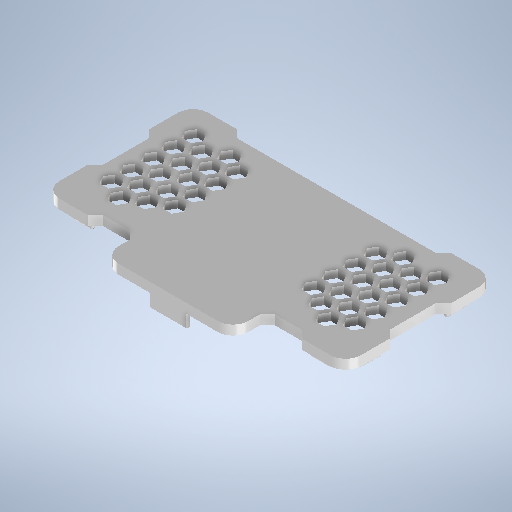
# Autodesk Inventor part: untitled22223333
Saved by Autodesk Inventor 2025.2 (Build 292293000, 293)
## iProperties
Created: 2025-03-09
Part Number: untitled22223333
Material: Ogólny
Document SubType Name: Modeling
Designer: admin
Density: 1 g/cm^3
Appearance: Domyślna
Author: admin
Autodesk Inventor part; units mm, degrees
(part 1 of 3)
ref_plane "YZ Plane" through (0, 0, 0) normal (1, 0, 0) x (0, 1, 0)
ref_plane "XZ Plane" through (0, 0, 0) normal (0, 1, 0) x (-1, 0, 0)
sketch "Szkic1" plane through (0, 0, 0) normal (0, 0, 1) x (1, 0, 0)
  line L0 (-39.2454, 11.2956) -> (-39.2454, -13.7044)
  line L1 (-36.2454, -16.7044) -> (28.7546, -16.7044)
  line L2 (31.7546, -13.7044) -> (31.7546, 11.2956)
  line L3 (-41.2454, 4.7956) -> (-41.2454, -7.2044)
  line L4 (-29.7595, -18.7044) -> (22.2546, -18.7044)
  line L5 (33.7546, -7.2044) -> (33.7546, 4.7956)
  line L6 (-43.2454, -9.2044) -> (-43.2454, -9.2044)
  line L7 (-43.2454, 6.7956) -> (-43.2454, 6.7956)
  line L8 (-39.2454, 6.7956) -> (-39.2454, -9.2044)
  line L9 (35.7546, -9.2044) -> (35.7546, -9.2044)
  line L10 (35.7546, 6.7956) -> (35.7546, 6.7956)
  line L11 (31.7546, 6.7956) -> (31.7546, -9.2044)
  line L12 (35.7546, 14.2956) -> (35.7546, 6.7956)
  line L13 (35.7546, -9.2044) -> (35.7546, -16.7044)
  line L14 (-43.2454, -16.7044) -> (-43.2454, -9.2044)
  line L15 (-43.2454, 6.7956) -> (-43.2454, 14.2956)
  line L16 (-31.7454, -20.7044) -> (-31.7454, -20.7044)
  line L17 (24.2546, -20.7044) -> (24.2546, -20.7044)
  line L18 (24.2546, 18.2956) -> (24.2546, 18.2956)
  line L19 (-31.7454, 18.2956) -> (-31.7454, 18.2956)
  line L20 (-39.2454, 18.2956) -> (-31.7454, 18.2956)
  line L21 (24.2546, 18.2956) -> (31.7546, 18.2956)
  line L22 (31.7546, -20.7044) -> (24.2546, -20.7044)
  line L23 (-31.7454, -20.7044) -> (-39.2454, -20.7044)
  line L24 (-31.7454, 18.2956) -> (-29.7454, 16.2956)
  line L25 (-43.2454, 6.7956) -> (-41.2454, 4.7956)
  line L26 (-43.2454, -9.2044) -> (-41.2454, -7.2044)
  line L27 (-31.7454, -20.7044) -> (-29.7595, -18.7044)
  line L28 (22.2546, -18.7044) -> (24.2546, -20.7044)
  line L29 (35.7546, -9.2044) -> (33.7546, -7.2044)
  line L30 (35.7546, 6.7956) -> (33.7546, 4.7956)
  line L31 (24.2546, 18.2956) -> (22.2546, 16.2956)
  line L32 (22.2546, 16.2956) -> (15.2546, 16.2956)
  line L33 (-22.7454, 16.2956) -> (-29.7454, 16.2956)
  arc A0 (-39.2454, 18.2956) -> (-43.2454, 14.2956) centre (-39.2454, 14.2956) ccw
  arc A1 (-43.2454, -16.7044) -> (-39.2454, -20.7044) centre (-39.2454, -16.7044) ccw
  arc A2 (31.7546, -20.7044) -> (35.7546, -16.7044) centre (31.7546, -16.7044) ccw
  arc A3 (35.7546, 14.2956) -> (31.7546, 18.2956) centre (31.7546, 14.2956) ccw
  line L34 (13.2546, 18.2956) -> (13.2546, 21.2956)
  line L35 (6.2546, 24.2956) -> (-13.7454, 24.2956)
  line L36 (-20.7454, 21.2956) -> (-20.7454, 18.2956)
  line L37 (-16.7454, 16.2956) -> (-16.7454, 21.2956)
  line L38 (9.2546, 16.2956) -> (9.2546, 21.2956)
  line L39 (13.2546, 18.2956) -> (15.2546, 16.2956)
  line L40 (-20.7454, 18.2956) -> (-22.7454, 16.2956)
  line L41 (-36.2454, 14.2956) -> (-19.5739, 14.2956)
  line L42 (-13.917, 24.2956) -> (6.4261, 24.2956)
  line L43 (9.2546, 25.2956) -> (-16.7454, 25.2956)
  arc A4 (-16.7454, 25.2956) -> (-20.7454, 21.2956) centre (-16.7454, 21.2956) ccw
  arc A5 (13.2546, 21.2956) -> (9.2546, 25.2956) centre (9.2546, 21.2956) ccw
  arc A6 (31.7546, 11.2956) -> (28.7546, 14.2956) centre (28.7546, 11.2956) ccw
  arc A7 (28.7546, -16.7044) -> (31.7546, -13.7044) centre (28.7546, -13.7044) ccw
  arc A8 (-39.2454, -13.7044) -> (-36.2454, -16.7044) centre (-36.2454, -13.7044) ccw
  arc A9 (-36.2454, 14.2956) -> (-39.2454, 11.2956) centre (-36.2454, 11.2956) ccw
  arc A10 (-13.7454, 24.2956) -> (-16.7454, 21.2956) centre (-13.7454, 21.2956) ccw
  arc A11 (9.2546, 21.2956) -> (6.2546, 24.2956) centre (6.2546, 21.2956) ccw
  line L44 (28.7546, 14.2956) -> (11.2546, 14.2956)
  line L45 (-18.7454, 14.2956) -> (-19.5739, 14.2956)
  arc A12 (-18.7454, 14.2956) -> (-16.7454, 16.2956) centre (-18.7454, 16.2956) ccw
  arc A13 (9.2546, 16.2956) -> (11.2546, 14.2956) centre (11.2546, 16.2956) ccw
  line L46 (-31.7454, -18.7044) -> (-38.2454, -18.7044) construction
  line L47 (-32.6454, -17.8044) -> (-37.3454, -17.8044)
  line L48 (-37.3454, -19.6044) -> (-32.6454, -19.6044)
  arc A14 (-32.6454, -19.6044) -> (-32.6454, -17.8044) centre (-32.6454, -18.7044) ccw
  arc A15 (-37.3454, -17.8044) -> (-37.3454, -19.6044) centre (-37.3454, -18.7044) ccw
  line L49 (-41.2454, -9.2044) -> (-41.2454, -15.7044) construction
  line L50 (-42.1454, -10.1044) -> (-42.1454, -14.8044)
  line L51 (-40.3454, -14.8044) -> (-40.3454, -10.1044)
  arc A16 (-40.3454, -10.1044) -> (-42.1454, -10.1044) centre (-41.2454, -10.1044) ccw
  arc A17 (-42.1454, -14.8044) -> (-40.3454, -14.8044) centre (-41.2454, -14.8044) ccw
  circle A18 centre (-40.2454, -17.7044) radius 1.5
  line L52 (24.2546, -18.7044) -> (30.7546, -18.7044) construction
  line L53 (25.1546, -17.8044) -> (29.8546, -17.8044)
  line L54 (29.8546, -19.6044) -> (25.1546, -19.6044)
  arc A19 (25.1546, -17.8044) -> (25.1546, -19.6044) centre (25.1546, -18.7044) ccw
  arc A20 (29.8546, -19.6044) -> (29.8546, -17.8044) centre (29.8546, -18.7044) ccw
  line L55 (33.7546, -9.2044) -> (33.7546, -15.7044) construction
  line L56 (34.6546, -10.1044) -> (34.6546, -14.8044)
  line L57 (32.8546, -14.8044) -> (32.8546, -10.1044)
  arc A21 (34.6546, -10.1044) -> (32.8546, -10.1044) centre (33.7546, -10.1044) ccw
  arc A22 (32.8546, -14.8044) -> (34.6546, -14.8044) centre (33.7546, -14.8044) ccw
  circle A23 centre (32.7546, -17.7044) radius 1.5
  line L58 (-43.2454, 6.7956) -> (-41.2454, 4.7956)
  line L59 (-31.7454, 16.2956) -> (-38.2454, 16.2956) construction
  line L60 (-32.6454, 15.3956) -> (-37.3454, 15.3956)
  line L61 (-37.3454, 17.1956) -> (-32.6454, 17.1956)
  arc A24 (-32.6454, 15.3956) -> (-32.6454, 17.1956) centre (-32.6454, 16.2956) ccw
  arc A25 (-37.3454, 17.1956) -> (-37.3454, 15.3956) centre (-37.3454, 16.2956) ccw
  line L62 (-41.2454, 6.7956) -> (-41.2454, 13.2956) construction
  line L63 (-42.1454, 7.6956) -> (-42.1454, 12.3956)
  line L64 (-40.3454, 12.3956) -> (-40.3454, 7.6956)
  arc A26 (-42.1454, 7.6956) -> (-40.3454, 7.6956) centre (-41.2454, 7.6956) ccw
  arc A27 (-40.3454, 12.3956) -> (-42.1454, 12.3956) centre (-41.2454, 12.3956) ccw
  circle A28 centre (-40.2454, 15.2956) radius 1.5
  circle A29 centre (32.7546, 15.2956) radius 1.5
  arc A30 (32.8546, 7.6956) -> (34.6546, 7.6956) centre (33.7546, 7.6956) ccw
  line L65 (34.6546, 7.6956) -> (34.6546, 12.3956)
  line L66 (33.7546, 6.7956) -> (33.7546, 13.2956) construction
  arc A31 (34.6546, 12.3956) -> (32.8546, 12.3956) centre (33.7546, 12.3956) ccw
  line L67 (32.8546, 12.3956) -> (32.8546, 7.6956)
  line L68 (24.2546, 16.2956) -> (30.7546, 16.2956) construction
  arc A32 (29.8546, 15.3956) -> (29.8546, 17.1956) centre (29.8546, 16.2956) ccw
  line L69 (29.8546, 17.1956) -> (25.1546, 17.1956)
  arc A33 (25.1546, 17.1956) -> (25.1546, 15.3956) centre (25.1546, 16.2956) ccw
  line L70 (25.1546, 15.3956) -> (29.8546, 15.3956)
  point P0 (0, 0)
  point P1 (33.7546, 6.7956)
  point P2 (-31.7454, 16.2956)
  point P3 (24.2546, -18.7044)
  point P4 (24.2546, 16.2956)
  point P5 (33.7546, -9.2044)
  point P6 (-41.2454, 6.7956)
  point P7 (-20.7454, 16.2956)
  point P8 (13.2546, 16.2956)
  point P9 (-16.7454, 24.2956)
  point P10 (24.2546, -20.7044)
  point P11 (35.7546, 6.7956)
  point P12 (24.2546, 18.2956)
  point P13 (-43.2454, 6.7956)
  point P14 (-34.9954, -18.7044)
  point P15 (-41.2454, -12.4544)
  point P16 (27.5046, -18.7044)
  point P17 (33.7546, -12.4544)
  point P18 (24.2546, 16.2956)
  point P19 (33.7546, 6.7956)
  point P20 (-34.9954, 16.2956)
  point P21 (-41.2454, 10.0456)
  point P22 (33.7546, 10.0456)
  point P23 (27.5046, 16.2956)
  dimension "d0" = 4
  dimension "d2" = 3
  dimension "d3" = 2
  dimension "d17" = 6.5
  dimension "d18" = 1.8
  dimension "d19" = 6.5
  dimension "d20" = 1.8
  dimension "d23" = 3
  dimension "d81" = 3
  dimension "d82" = 3
  dimension "d83" = 3
  constraints: 158 end point, 76 point on circle, 40 point on line, 37 tangent, 34 centre point, 25 parallel, 9 perpendicular, 8 equal radius, 4 horizontal, 2 midpoint, 1 vertical
  measures "d0" radius of A0
  measures "d2" radius of A10
  measures "d3" radius of A12
  measures "d17" distance of L46.start L46.end
  measures "d18" diameter of A15
  measures "d19" distance of L49.start L49.end
  measures "d20" diameter of A17
  measures "d23" diameter of A18
  measures "d81" diameter of A28
  measures "d82" diameter of A29
  measures "d83" diameter of A23
extrude "Wyciągnięcie proste1" add sketch "Szkic1" along normal blind 2.5 contours A9 L41 L45 A12 L37 A10 L35 A11 L38 A13 L44 A6 L2 A7 L1 A8 L0 | L25 L15 A0 L20 L24 L33 L40 L36 A4 L43 A5 L34 L39 L32 L31 L21 A3 L12 L30 L5 L29 L13 A2 L22 L28 L4 L27 L23 A1 L14 L26 L3 | A14 L48 A15 L47 | A16 L51 A17 L50 | A18 | L53 A20 L54 A19 | L56 A22 L57 A21 | A23 | L60 A25 L61 A24 | L63 A27 L64 A26 | A28 | A29 | L67 A31 L65 A30 | L70 A33 L69 A32
extrude "Wyciągnięcie proste4" cut sketch "Szkic1" along normal blind 1.6 contours A18 | A23 | A28 | A29
sketch "Szkic4" plane through (0, 0, 0) normal (0, 0, -1) x (-1, 0, 0)
  line L0 (-9.2546, 25.2956) -> (16.7454, 25.2956) projected
  line L1 (-0.9446, 24.2956) -> (8.4354, 24.2956)
  line L2 (8.4354, 24.2956) -> (8.4354, 25.2956)
  line L3 (8.4354, 26.2956) -> (-0.9446, 24.2956) construction
  line L4 (-0.9446, 26.2956) -> (8.4354, 24.2956) construction
  line L5 (8.4354, 25.2956) -> (-0.9446, 25.2956)
  line L6 (-0.9446, 24.2956) -> (-0.9446, 25.2956)
  line L7 (8.4354, 25.2956) -> (-0.9446, 25.2956)
  point P0 (0, 0)
  constraints: 14 end point, 1 collinear, 1 perpendicular, 1 point on line
extrude "Wyciągnięcie proste6" add sketch "Szkic4" along normal blind 3.5
sketch "Szkic5" plane through (0, 0, 0) normal (0, 0, -1) x (-1, 0, 0)
  line L0 (8.4425, -20.7044) -> (-0.9375, -20.7044)
  line L1 (-0.9375, -20.7044) -> (-0.9375, -16.7044)
  line L2 (-0.9375, -16.7044) -> (8.4425, -16.7044)
  line L3 (8.4425, -16.7044) -> (8.4425, -20.7044)
  line L4 (29.7595, -18.7044) -> (-22.2546, -18.7044) projected
  line L5 (8.4425, -20.7044) -> (-0.9375, -16.7044) construction
  line L6 (-0.9375, -20.7044) -> (8.4425, -16.7044) construction
  line L7 (8.4425, -18.7044) -> (-0.9375, -18.7044)
  point P0 (0, 0)
  point P1 (3.7525, -18.7044)
  dimension "d32" = 9.38
  dimension "d33" = 4
  constraints: 14 end point, 5 midpoint, 2 parallel, 2 point on line, 1 horizontal, 1 perpendicular
  measures "d32" distance of L1.end L2.end
  measures "d33" distance of L0.end L1.end
extrude "Wyciągnięcie proste7" add sketch "Szkic5" along normal blind 4 contours L4 L1 L2 L3
ref_plane "Płaszczyzna konstrukcyjna2" through (0, 0, -2) normal (0, 0, -1) x (-1, 0, 0)
sketch "Szkic7" plane through (0, 0, -2) normal (0, 0, -1) x (-1, 0, 0)
  arc A0 (-25.1546, 15.6456) -> (-25.1546, 16.9456) centre (-25.1546, 16.2956) ccw projected
  arc A1 (-29.8546, 16.9456) -> (-29.8546, 15.6456) centre (-29.8546, 16.2956) ccw projected
  line L0 (-25.1546, 16.2956) -> (-25.2546, 16.2956)
  line L1 (-29.8546, 16.2956) -> (-29.7546, 16.2956)
  arc A2 (-25.2546, 15.3956) -> (-25.2546, 17.1956) centre (-25.2546, 16.2956) ccw
  line L2 (-25.1546, 15.3956) -> (-29.8546, 15.3956) projected
  arc A3 (-29.7546, 17.1956) -> (-29.7546, 15.3956) centre (-29.7546, 16.2956) ccw
  line L3 (-25.2546, 15.3956) -> (-29.7546, 15.3956)
  line L4 (-25.2546, 17.1956) -> (-29.7546, 17.1956)
  line L5 (-25.1546, 17.1956) -> (-29.8546, 17.1956) projected
  line L6 (-33.7546, 12.3956) -> (-33.7546, 12.2956)
  arc A4 (-34.4046, 7.6956) -> (-33.1046, 7.6956) centre (-33.7546, 7.6956) ccw projected
  line L7 (-33.7546, 7.6956) -> (-33.7546, 7.7956)
  arc A5 (-32.8546, 12.2956) -> (-34.6546, 12.2956) centre (-33.7546, 12.2956) ccw
  line L8 (-34.6546, 7.6956) -> (-34.6546, 12.3956) projected
  arc A6 (-34.6546, 7.7956) -> (-32.8546, 7.7956) centre (-33.7546, 7.7956) ccw
  line L9 (-32.8546, 12.3956) -> (-32.8546, 7.6956) projected
  line L10 (-32.8546, 7.7956) -> (-32.8546, 12.2956)
  line L11 (-34.6546, 12.2956) -> (-34.6546, 7.7956)
  line L12 (-33.7546, -7.2044) -> (-33.7546, 4.7956) projected
  line L13 (-33.7546, -1.2044) -> (-29.2219, -1.2044)
  line L14 (8.4354, 25.2956) -> (-0.9446, 25.2956) projected
  line L15 (3.7454, 25.2956) -> (3.7454, 21.1708)
  arc A7 (-25.1546, -19.3544) -> (-25.1546, -18.0544) centre (-25.1546, -18.7044) ccw
  arc A8 (-29.8546, -18.0544) -> (-29.8546, -19.3544) centre (-29.8546, -18.7044) ccw
  line L16 (-25.1546, -18.7044) -> (-25.2546, -18.7044)
  line L17 (-29.8546, -18.7044) -> (-29.7546, -18.7044)
  arc A9 (-25.2546, -19.6044) -> (-25.2546, -17.8044) centre (-25.2546, -18.7044) ccw
  line L18 (-25.1546, -17.8044) -> (-29.8546, -17.8044)
  arc A10 (-29.7546, -17.8044) -> (-29.7546, -19.6044) centre (-29.7546, -18.7044) ccw
  line L19 (-25.2546, -17.8044) -> (-29.7546, -17.8044)
  line L20 (-25.2546, -19.6044) -> (-29.7546, -19.6044)
  line L21 (-25.1546, -19.6044) -> (-29.8546, -19.6044)
  line L22 (-33.7546, -14.8044) -> (-33.7546, -14.7044)
  arc A11 (-33.1046, -10.1044) -> (-34.4046, -10.1044) centre (-33.7546, -10.1044) ccw
  line L23 (-33.7546, -10.1044) -> (-33.7546, -10.2044)
  arc A12 (-34.6546, -14.7044) -> (-32.8546, -14.7044) centre (-33.7546, -14.7044) ccw
  line L24 (-34.6546, -10.1044) -> (-34.6546, -14.8044)
  arc A13 (-32.8546, -10.2044) -> (-34.6546, -10.2044) centre (-33.7546, -10.2044) ccw
  line L25 (-32.8546, -14.8044) -> (-32.8546, -10.1044)
  line L26 (-32.8546, -10.2044) -> (-32.8546, -14.7044)
  line L27 (-34.6546, -14.7044) -> (-34.6546, -10.2044)
  arc A14 (32.6454, 16.9456) -> (32.6454, 15.6456) centre (32.6454, 16.2956) ccw
  arc A15 (37.3454, 15.6456) -> (37.3454, 16.9456) centre (37.3454, 16.2956) ccw
  line L28 (32.6454, 16.2956) -> (32.7454, 16.2956)
  line L29 (37.3454, 16.2956) -> (37.2454, 16.2956)
  arc A16 (32.7454, 17.1956) -> (32.7454, 15.3956) centre (32.7454, 16.2956) ccw
  line L30 (32.6454, 15.3956) -> (37.3454, 15.3956)
  arc A17 (37.2454, 15.3956) -> (37.2454, 17.1956) centre (37.2454, 16.2956) ccw
  line L31 (32.7454, 15.3956) -> (37.2454, 15.3956)
  line L32 (32.7454, 17.1956) -> (37.2454, 17.1956)
  line L33 (32.6454, 17.1956) -> (37.3454, 17.1956)
  line L34 (41.2454, 12.3956) -> (41.2454, 12.2956)
  arc A18 (40.5954, 7.6956) -> (41.8954, 7.6956) centre (41.2454, 7.6956) ccw
  line L35 (41.2454, 7.6956) -> (41.2454, 7.7956)
  arc A19 (42.1454, 12.2956) -> (40.3454, 12.2956) centre (41.2454, 12.2956) ccw
  line L36 (42.1454, 7.6956) -> (42.1454, 12.3956)
  arc A20 (40.3454, 7.7956) -> (42.1454, 7.7956) centre (41.2454, 7.7956) ccw
  line L37 (40.3454, 12.3956) -> (40.3454, 7.6956)
  line L38 (40.3454, 7.7956) -> (40.3454, 12.2956)
  line L39 (42.1454, 12.2956) -> (42.1454, 7.7956)
  line L40 (41.2454, -7.2044) -> (41.2454, 4.7956)
  arc A21 (32.6454, -18.0544) -> (32.6454, -19.3544) centre (32.6454, -18.7044) ccw
  arc A22 (32.7454, -17.8044) -> (32.7454, -19.6044) centre (32.7454, -18.7044) ccw
  line L41 (32.7454, -19.6044) -> (37.2454, -19.6044)
  line L42 (32.6454, -19.6044) -> (37.3454, -19.6044)
  line L43 (37.3454, -18.7044) -> (37.2454, -18.7044)
  line L44 (32.7454, -17.8044) -> (37.2454, -17.8044)
  line L45 (32.6454, -17.8044) -> (37.3454, -17.8044)
  arc A23 (37.3454, -19.3544) -> (37.3454, -18.0544) centre (37.3454, -18.7044) ccw
  arc A24 (37.2454, -19.6044) -> (37.2454, -17.8044) centre (37.2454, -18.7044) ccw
  line L46 (32.6454, -18.7044) -> (32.7454, -18.7044)
  line L47 (41.2454, -14.8044) -> (41.2454, -14.7044)
  line L48 (40.3454, -10.2044) -> (40.3454, -14.7044)
  line L49 (40.3454, -14.8044) -> (40.3454, -10.1044)
  arc A25 (40.3454, -14.7044) -> (42.1454, -14.7044) centre (41.2454, -14.7044) ccw
  line L50 (41.2454, -10.1044) -> (41.2454, -10.2044)
  line L51 (42.1454, -14.7044) -> (42.1454, -10.2044)
  line L52 (42.1454, -10.1044) -> (42.1454, -14.8044)
  arc A26 (42.1454, -10.2044) -> (40.3454, -10.2044) centre (41.2454, -10.2044) ccw
  arc A27 (41.8954, -10.1044) -> (40.5954, -10.1044) centre (41.2454, -10.1044) ccw
  point P0 (0, 0)
  dimension "d43" = 0.1
  dimension "d44" = 0.1
  dimension "d45" = 0.1
  dimension "d46" = 0.1
  constraints: 104 symmetric about line, 94 end point, 50 point on circle, 28 point on line, 25 centre point, 16 coincident, 4 tangent, 3 horizontal, 3 vertical, 2 midpoint, 21 other
  measures "d43" distance of L0.start L0.end
  measures "d44" distance of L1.start L1.end
  measures "d45" distance of L6.start L6.end
  measures "d46" distance of L7.start L7.end
extrude "Wyciągnięcie proste8" add sketch "Szkic7" along normal blind 2 from surface at -2
sketch "Szkic10" plane through (0, 0, 2.5) normal (0, 0, 1) x (1, 0, 0)
  point P0 (0, 0)
sketch "Szkic11" plane through (0, 0, 2.5) normal (0, 0, 1) x (1, 0, 0)
  point P0 (0, 0)
sketch "Szkic12" plane through (0, 0, -2) normal (0, 0, -1) x (-1, 0, 0)
  arc A0 (-29.7546, 17.1956) -> (-29.7546, 15.3956) centre (-29.7546, 16.2956) ccw projected
  line L0 (-29.7546, 17.1956) -> (-25.2546, 17.1956) projected
  arc A1 (-25.2546, 15.3956) -> (-25.2546, 17.1956) centre (-25.2546, 16.2956) ccw projected
  line L1 (-25.2546, 15.3956) -> (-29.7546, 15.3956) projected
  line L2 (32.7454, -17.8044) -> (37.2454, -17.8044) projected
  arc A2 (37.2454, -19.6044) -> (37.2454, -17.8044) centre (37.2454, -18.7044) ccw projected
  line L3 (37.2454, -19.6044) -> (32.7454, -19.6044) projected
  arc A3 (32.7454, -17.8044) -> (32.7454, -19.6044) centre (32.7454, -18.7044) ccw projected
  line L4 (-25.2546, -19.6044) -> (-29.7546, -19.6044) projected
  arc A4 (-29.7546, -17.8044) -> (-29.7546, -19.6044) centre (-29.7546, -18.7044) ccw projected
  line L5 (-29.7546, -17.8044) -> (-25.2546, -17.8044) projected
  arc A5 (-25.2546, -19.6044) -> (-25.2546, -17.8044) centre (-25.2546, -18.7044) ccw projected
  arc A6 (32.7454, 17.1956) -> (32.7454, 15.3956) centre (32.7454, 16.2956) ccw projected
  line L6 (32.7454, 17.1956) -> (37.2454, 17.1956) projected
  arc A7 (37.2454, 15.3956) -> (37.2454, 17.1956) centre (37.2454, 16.2956) ccw projected
  line L7 (37.2454, 15.3956) -> (32.7454, 15.3956) projected
  arc A8 (-32.8546, 12.2956) -> (-34.6546, 12.2956) centre (-33.7546, 12.2956) ccw projected
  line L8 (-32.8546, 12.2956) -> (-32.8546, 7.7956) projected
  arc A9 (-34.6546, 7.7956) -> (-32.8546, 7.7956) centre (-33.7546, 7.7956) ccw projected
  line L9 (-34.6546, 7.7956) -> (-34.6546, 12.2956) projected
  line L10 (42.1454, -10.2044) -> (42.1454, -14.7044) projected
  arc A10 (40.3454, -14.7044) -> (42.1454, -14.7044) centre (41.2454, -14.7044) ccw projected
  line L11 (40.3454, -14.7044) -> (40.3454, -10.2044) projected
  arc A11 (42.1454, -10.2044) -> (40.3454, -10.2044) centre (41.2454, -10.2044) ccw projected
  line L12 (-34.6546, -14.7044) -> (-34.6546, -10.2044) projected
  arc A12 (-32.8546, -10.2044) -> (-34.6546, -10.2044) centre (-33.7546, -10.2044) ccw projected
  line L13 (-32.8546, -10.2044) -> (-32.8546, -14.7044) projected
  arc A13 (-34.6546, -14.7044) -> (-32.8546, -14.7044) centre (-33.7546, -14.7044) ccw projected
  arc A14 (42.1454, 12.2956) -> (40.3454, 12.2956) centre (41.2454, 12.2956) ccw projected
  line L14 (42.1454, 12.2956) -> (42.1454, 7.7956) projected
  arc A15 (40.3454, 7.7956) -> (42.1454, 7.7956) centre (41.2454, 7.7956) ccw projected
  line L15 (40.3454, 7.7956) -> (40.3454, 12.2956) projected
  line L16 (-0.9375, -16.7044) -> (8.4425, -16.7044) projected
  line L17 (8.4425, -16.7044) -> (8.4425, -18.7044) projected
  line L18 (8.4425, -18.7044) -> (-0.9375, -18.7044) projected
  line L19 (-0.9375, -18.7044) -> (-0.9375, -16.7044) projected
  line L20 (-0.9446, 24.2956) -> (-0.9446, 25.2956) projected
  line L21 (-0.9446, 25.2956) -> (8.4354, 25.2956) projected
  line L22 (8.4354, 25.2956) -> (8.4354, 24.2956) projected
  line L23 (8.4354, 24.2956) -> (-0.9446, 24.2956) projected
  point P0 (0, 0)
sketch "Szkic13" plane through (0, 0, 2.5) normal (0, 0, 1) x (1, 0, 0)
  line L0 (50.8212, 20.6161) -> (50.8393, 20.6161)
  spline S0 degree 3 poles (59.7766, 12.8398) (60.2327, 11.0243) (60.1356, 9.6953) (59.6392, 8.6942) knots 0 0 0 0 1 1 1 1
  line L1 (59.7766, 12.8398) -> (60.2327, 11.0243) construction
  line L2 (60.2327, 11.0243) -> (60.1356, 9.6953) construction
  line L3 (60.1356, 9.6953) -> (59.6392, 8.6942) construction
  spline S1 degree 3 poles (59.6392, 8.6942) (59.0896, 7.5838) (58.0818, 6.9244) (56.9635, 6.413) knots 0 0 0 0 1 1 1 1
  line L4 (59.6392, 8.6942) -> (59.0896, 7.5838) construction
  line L5 (59.0896, 7.5838) -> (58.0818, 6.9244) construction
  line L6 (58.0818, 6.9244) -> (56.9635, 6.413) construction
  spline S2 degree 3 poles (56.9635, 6.413) (54.7944, 5.4206) (52.1806, 4.9088) (50.9724, 2.9978) knots 0 0 0 0 1 1 1 1
  line L7 (56.9635, 6.413) -> (54.7944, 5.4206) construction
  line L8 (54.7944, 5.4206) -> (52.1806, 4.9088) construction
  line L9 (52.1806, 4.9088) -> (50.9724, 2.9978) construction
  spline S3 degree 3 poles (50.9724, 2.9978) (62.5222, 3.9472) (61.4236, 10.5113) (59.7766, 12.8394) knots 0 0 0 0 1 1 1 1
  line L10 (50.9724, 2.9978) -> (62.5222, 3.9472) construction
  line L11 (62.5222, 3.9472) -> (61.4236, 10.5113) construction
  line L12 (61.4236, 10.5113) -> (59.7766, 12.8394) construction
  spline S4 degree 3 poles (59.3216, 12.2021) (59.12, 11.2579) (58.3272, 10.3333) (56.1573, 9.305) knots 0 0 0 0 1 1 1 1
  line L13 (59.3216, 12.2021) -> (59.12, 11.2579) construction
  line L14 (59.12, 11.2579) -> (58.3272, 10.3333) construction
  line L15 (58.3272, 10.3333) -> (56.1573, 9.305) construction
  spline S5 degree 3 poles (56.1573, 9.305) (54.4219, 8.4831) (51.833, 6.4896) (50.867, 3.858) knots 0 0 0 0 1 1 1 1
  line L16 (56.1573, 9.305) -> (54.4219, 8.4831) construction
  line L17 (54.4219, 8.4831) -> (51.833, 6.4896) construction
  line L18 (51.833, 6.4896) -> (50.867, 3.858) construction
  spline S6 degree 3 poles (50.867, 3.858) (52.3353, 5.6077) (54.835, 6.1017) (56.7256, 6.9662) knots 0 0 0 0 1 1 1 1
  line L19 (50.867, 3.858) -> (52.3353, 5.6077) construction
  line L20 (52.3353, 5.6077) -> (54.835, 6.1017) construction
  line L21 (54.835, 6.1017) -> (56.7256, 6.9662) construction
  spline S7 degree 3 poles (56.7256, 6.9662) (57.7914, 7.4536) (58.6559, 8.0395) (59.116, 8.9692) knots 0 0 0 0 1 1 1 1
  line L22 (56.7256, 6.9662) -> (57.7914, 7.4536) construction
  line L23 (57.7914, 7.4536) -> (58.6559, 8.0395) construction
  line L24 (58.6559, 8.0395) -> (59.116, 8.9692) construction
  spline S8 degree 3 poles (59.116, 8.9692) (59.4917, 9.7264) (59.6187, 10.7449) (59.3212, 12.2017) knots 0 0 0 0 1 1 1 1
  line L25 (59.116, 8.9692) -> (59.4917, 9.7264) construction
  line L26 (59.4917, 9.7264) -> (59.6187, 10.7449) construction
  line L27 (59.6187, 10.7449) -> (59.3212, 12.2017) construction
  line L28 (59.7766, 12.8394) -> (59.7766, 12.8398)
  line L29 (59.3212, 12.2017) -> (59.3216, 12.2021)
  spline S9 degree 3 poles (50.3023, 13.6049) (49.8209, 13.0892) (49.4109, 12.519) (49.0448, 11.9157) knots 0 0 0 0 1 1 1 1
  line L30 (50.3023, 13.6049) -> (49.8209, 13.0892) construction
  line L31 (49.8209, 13.0892) -> (49.4109, 12.519) construction
  line L32 (49.4109, 12.519) -> (49.0448, 11.9157) construction
  spline S10 degree 3 poles (49.0448, 11.9157) (49.0438, 11.6548) (49.0843, 11.3881) (49.1994, 11.1123) knots 0 0 0 0 1 1 1 1
  line L33 (49.0448, 11.9157) -> (49.0438, 11.6548) construction
  line L34 (49.0438, 11.6548) -> (49.0843, 11.3881) construction
  line L35 (49.0843, 11.3881) -> (49.1994, 11.1123) construction
  spline S11 degree 3 poles (49.1994, 11.1123) (49.4192, 10.6186) (49.7266, 10.3617) (50.1153, 10.3278) knots 0 0 0 0 1 1 1 1
  line L36 (49.1994, 11.1123) -> (49.4192, 10.6186) construction
  line L37 (49.4192, 10.6186) -> (49.7266, 10.3617) construction
  line L38 (49.7266, 10.3617) -> (50.1153, 10.3278) construction
  spline S12 degree 3 poles (50.1153, 10.3278) (49.8683, 10.6328) (49.7542, 10.9264) (49.7148, 11.2137) knots 0 0 0 0 1 1 1 1
  line L39 (50.1153, 10.3278) -> (49.8683, 10.6328) construction
  line L40 (49.8683, 10.6328) -> (49.7542, 10.9264) construction
  line L41 (49.7542, 10.9264) -> (49.7148, 11.2137) construction
  spline S13 degree 3 poles (49.7148, 11.2137) (49.6943, 11.3952) (50.0995, 12.3237) (50.5371, 12.5967) knots 0 0 0 0 1 1 1 1
  line L42 (49.7148, 11.2137) -> (49.6943, 11.3952) construction
  line L43 (49.6943, 11.3952) -> (50.0995, 12.3237) construction
  line L44 (50.0995, 12.3237) -> (50.5371, 12.5967) construction
  spline S14 degree 3 poles (50.5371, 12.5967) (50.676, 12.6057) (51.434, 12.3734) (52.3657, 12.0735) knots 0 0 0 0 1 1 1 1
  line L45 (50.5371, 12.5967) -> (50.676, 12.6057) construction
  line L46 (50.676, 12.6057) -> (51.434, 12.3734) construction
  line L47 (51.434, 12.3734) -> (52.3657, 12.0735) construction
  line L48 (51.876, 12.8086) -> (51.4656, 13.2415)
  line L49 (51.4656, 13.2415) -> (51.2237, 13.4956)
  line L50 (51.2237, 13.4956) -> (50.3023, 13.6049)
  spline S15 degree 3 poles (56.4825, 21.5532) (56.4119, 21.6503) (56.3626, 21.7776) (56.3625, 21.7778) knots 0 0 0 0 1 1 1 1
  line L51 (56.4825, 21.5532) -> (56.4119, 21.6503) construction
  line L52 (56.4119, 21.6503) -> (56.3625, 21.7778) construction
  line L53 (56.3625, 21.7778) -> (56.3625, 21.7778) construction
  spline S16 degree 3 poles (56.3625, 21.7778) (56.3625, 21.7776) (56.3136, 21.6503) (56.2426, 21.554) knots 0 0 0 0 1 1 1 1
  line L54 (56.3625, 21.7778) -> (56.3625, 21.7778) construction
  line L55 (56.3625, 21.7778) -> (56.3136, 21.6503) construction
  line L56 (56.3136, 21.6503) -> (56.2426, 21.554) construction
  spline S17 degree 3 poles (56.2426, 21.554) (56.2055, 21.5027) (56.1601, 21.4546) (56.1601, 21.3863) knots 0 0 0 0 1 1 1 1
  line L57 (56.2426, 21.554) -> (56.2055, 21.5027) construction
  line L58 (56.2055, 21.5027) -> (56.1601, 21.4546) construction
  line L59 (56.1601, 21.4546) -> (56.1601, 21.3863) construction
  spline S18 degree 3 poles (56.1601, 21.3863) (56.1601, 21.318) (56.2047, 21.2699) (56.2422, 21.219) knots 0 0 0 0 1 1 1 1
  line L60 (56.1601, 21.3863) -> (56.1601, 21.318) construction
  line L61 (56.1601, 21.318) -> (56.2047, 21.2699) construction
  line L62 (56.2047, 21.2699) -> (56.2422, 21.219) construction
  spline S19 degree 3 poles (56.2422, 21.219) (56.3128, 21.1215) (56.3625, 20.9946) (56.3625, 20.9945) knots 0 0 0 0 1 1 1 1
  line L63 (56.2422, 21.219) -> (56.3128, 21.1215) construction
  line L64 (56.3128, 21.1215) -> (56.3625, 20.9945) construction
  line L65 (56.3625, 20.9945) -> (56.3625, 20.9945) construction
  spline S20 degree 3 poles (56.3625, 20.9945) (56.3626, 20.9946) (56.411, 21.1216) (56.4821, 21.2186) knots 0 0 0 0 1 1 1 1
  line L66 (56.3625, 20.9945) -> (56.3625, 20.9945) construction
  line L67 (56.3625, 20.9945) -> (56.411, 21.1216) construction
  line L68 (56.411, 21.1216) -> (56.4821, 21.2186) construction
  spline S21 degree 3 poles (56.4821, 21.2186) (56.5192, 21.2695) (56.5642, 21.3176) (56.5642, 21.3863) knots 0 0 0 0 1 1 1 1
  line L69 (56.4821, 21.2186) -> (56.5192, 21.2695) construction
  line L70 (56.5192, 21.2695) -> (56.5642, 21.3176) construction
  line L71 (56.5642, 21.3176) -> (56.5642, 21.3863) construction
  spline S22 degree 3 poles (56.5642, 21.3863) (56.5642, 21.455) (56.52, 21.5023) (56.4825, 21.5532) knots 0 0 0 0 1 1 1 1
  line L72 (56.5642, 21.3863) -> (56.5642, 21.455) construction
  line L73 (56.5642, 21.455) -> (56.52, 21.5023) construction
  line L74 (56.52, 21.5023) -> (56.4825, 21.5532) construction
  line L75 (52.3657, 12.0735) -> (52.6123, 12.0325)
  line L76 (52.6123, 12.0325) -> (51.876, 12.8086)
  spline S23 degree 3 poles (56.4825, 21.5532) (56.4119, 21.6503) (56.3626, 21.7776) (56.3625, 21.7778) knots 0 0 0 0 1 1 1 1
  line L77 (56.4825, 21.5532) -> (56.4119, 21.6503) construction
  line L78 (56.4119, 21.6503) -> (56.3625, 21.7778) construction
  line L79 (56.3625, 21.7778) -> (56.3625, 21.7778) construction
  spline S24 degree 3 poles (56.3625, 21.7778) (56.3625, 21.7776) (56.3136, 21.6503) (56.2426, 21.554) knots 0 0 0 0 1 1 1 1
  line L80 (56.3625, 21.7778) -> (56.3625, 21.7778) construction
  line L81 (56.3625, 21.7778) -> (56.3136, 21.6503) construction
  line L82 (56.3136, 21.6503) -> (56.2426, 21.554) construction
  spline S25 degree 3 poles (56.2426, 21.554) (56.2055, 21.5027) (56.1601, 21.4546) (56.1601, 21.3863) knots 0 0 0 0 1 1 1 1
  line L83 (56.2426, 21.554) -> (56.2055, 21.5027) construction
  line L84 (56.2055, 21.5027) -> (56.1601, 21.4546) construction
  line L85 (56.1601, 21.4546) -> (56.1601, 21.3863) construction
  spline S26 degree 3 poles (56.1601, 21.3863) (56.1601, 21.318) (56.2047, 21.2699) (56.2422, 21.219) knots 0 0 0 0 1 1 1 1
  line L86 (56.1601, 21.3863) -> (56.1601, 21.318) construction
  line L87 (56.1601, 21.318) -> (56.2047, 21.2699) construction
  line L88 (56.2047, 21.2699) -> (56.2422, 21.219) construction
  spline S27 degree 3 poles (56.2422, 21.219) (56.3128, 21.1215) (56.3625, 20.9946) (56.3625, 20.9945) knots 0 0 0 0 1 1 1 1
  line L89 (56.2422, 21.219) -> (56.3128, 21.1215) construction
  line L90 (56.3128, 21.1215) -> (56.3625, 20.9945) construction
  line L91 (56.3625, 20.9945) -> (56.3625, 20.9945) construction
  spline S28 degree 3 poles (56.3625, 20.9945) (56.3626, 20.9946) (56.411, 21.1216) (56.4821, 21.2186) knots 0 0 0 0 1 1 1 1
  line L92 (56.3625, 20.9945) -> (56.3625, 20.9945) construction
  line L93 (56.3625, 20.9945) -> (56.411, 21.1216) construction
  line L94 (56.411, 21.1216) -> (56.4821, 21.2186) construction
  spline S29 degree 3 poles (56.4821, 21.2186) (56.5192, 21.2695) (56.5642, 21.3176) (56.5642, 21.3863) knots 0 0 0 0 1 1 1 1
  line L95 (56.4821, 21.2186) -> (56.5192, 21.2695) construction
  line L96 (56.5192, 21.2695) -> (56.5642, 21.3176) construction
  line L97 (56.5642, 21.3176) -> (56.5642, 21.3863) construction
  spline S30 degree 3 poles (56.5642, 21.3863) (56.5642, 21.455) (56.52, 21.5023) (56.4825, 21.5532) knots 0 0 0 0 1 1 1 1
  line L98 (56.5642, 21.3863) -> (56.5642, 21.455) construction
  line L99 (56.5642, 21.455) -> (56.52, 21.5023) construction
  line L100 (56.52, 21.5023) -> (56.4825, 21.5532) construction
  spline S31 degree 3 poles (56.4825, 21.5532) (56.4119, 21.6503) (56.3626, 21.7776) (56.3625, 21.7778) knots 0 0 0 0 1 1 1 1
  line L101 (56.4825, 21.5532) -> (56.4119, 21.6503) construction
  line L102 (56.4119, 21.6503) -> (56.3625, 21.7778) construction
  line L103 (56.3625, 21.7778) -> (56.3625, 21.7778) construction
  spline S32 degree 3 poles (56.3625, 21.7778) (56.3625, 21.7776) (56.3136, 21.6503) (56.2426, 21.554) knots 0 0 0 0 1 1 1 1
  line L104 (56.3625, 21.7778) -> (56.3625, 21.7778) construction
  line L105 (56.3625, 21.7778) -> (56.3136, 21.6503) construction
  line L106 (56.3136, 21.6503) -> (56.2426, 21.554) construction
  spline S33 degree 3 poles (56.2426, 21.554) (56.2055, 21.5027) (56.1601, 21.4546) (56.1601, 21.3863) knots 0 0 0 0 1 1 1 1
  line L107 (56.2426, 21.554) -> (56.2055, 21.5027) construction
  line L108 (56.2055, 21.5027) -> (56.1601, 21.4546) construction
  line L109 (56.1601, 21.4546) -> (56.1601, 21.3863) construction
  spline S34 degree 3 poles (56.1601, 21.3863) (56.1601, 21.318) (56.2047, 21.2699) (56.2422, 21.219) knots 0 0 0 0 1 1 1 1
  line L110 (56.1601, 21.3863) -> (56.1601, 21.318) construction
  line L111 (56.1601, 21.318) -> (56.2047, 21.2699) construction
  line L112 (56.2047, 21.2699) -> (56.2422, 21.219) construction
  spline S35 degree 3 poles (56.2422, 21.219) (56.3128, 21.1215) (56.3625, 20.9946) (56.3625, 20.9945) knots 0 0 0 0 1 1 1 1
  line L113 (56.2422, 21.219) -> (56.3128, 21.1215) construction
  line L114 (56.3128, 21.1215) -> (56.3625, 20.9945) construction
  line L115 (56.3625, 20.9945) -> (56.3625, 20.9945) construction
  spline S36 degree 3 poles (56.3625, 20.9945) (56.3626, 20.9946) (56.411, 21.1216) (56.4821, 21.2186) knots 0 0 0 0 1 1 1 1
  line L116 (56.3625, 20.9945) -> (56.3625, 20.9945) construction
  line L117 (56.3625, 20.9945) -> (56.411, 21.1216) construction
  line L118 (56.411, 21.1216) -> (56.4821, 21.2186) construction
  spline S37 degree 3 poles (56.4821, 21.2186) (56.5192, 21.2695) (56.5642, 21.3176) (56.5642, 21.3863) knots 0 0 0 0 1 1 1 1
  line L119 (56.4821, 21.2186) -> (56.5192, 21.2695) construction
  line L120 (56.5192, 21.2695) -> (56.5642, 21.3176) construction
  line L121 (56.5642, 21.3176) -> (56.5642, 21.3863) construction
  spline S38 degree 3 poles (56.5642, 21.3863) (56.5642, 21.455) (56.52, 21.5023) (56.4825, 21.5532) knots 0 0 0 0 1 1 1 1
  line L122 (56.5642, 21.3863) -> (56.5642, 21.455) construction
  line L123 (56.5642, 21.455) -> (56.52, 21.5023) construction
  line L124 (56.52, 21.5023) -> (56.4825, 21.5532) construction
  spline S39 degree 3 poles (56.4825, 21.5532) (56.4119, 21.6503) (56.3626, 21.7776) (56.3625, 21.7778) knots 0 0 0 0 1 1 1 1
  line L125 (56.4825, 21.5532) -> (56.4119, 21.6503) construction
  line L126 (56.4119, 21.6503) -> (56.3625, 21.7778) construction
  line L127 (56.3625, 21.7778) -> (56.3625, 21.7778) construction
  spline S40 degree 3 poles (56.3625, 21.7778) (56.3625, 21.7776) (56.3136, 21.6503) (56.2426, 21.554) knots 0 0 0 0 1 1 1 1
  line L128 (56.3625, 21.7778) -> (56.3625, 21.7778) construction
  line L129 (56.3625, 21.7778) -> (56.3136, 21.6503) construction
  line L130 (56.3136, 21.6503) -> (56.2426, 21.554) construction
  spline S41 degree 3 poles (56.2426, 21.554) (56.2055, 21.5027) (56.1601, 21.4546) (56.1601, 21.3863) knots 0 0 0 0 1 1 1 1
  line L131 (56.2426, 21.554) -> (56.2055, 21.5027) construction
  line L132 (56.2055, 21.5027) -> (56.1601, 21.4546) construction
  line L133 (56.1601, 21.4546) -> (56.1601, 21.3863) construction
  spline S42 degree 3 poles (56.1601, 21.3863) (56.1601, 21.318) (56.2047, 21.2699) (56.2422, 21.219) knots 0 0 0 0 1 1 1 1
  line L134 (56.1601, 21.3863) -> (56.1601, 21.318) construction
  line L135 (56.1601, 21.318) -> (56.2047, 21.2699) construction
  line L136 (56.2047, 21.2699) -> (56.2422, 21.219) construction
  spline S43 degree 3 poles (56.2422, 21.219) (56.3128, 21.1215) (56.3625, 20.9946) (56.3625, 20.9945) knots 0 0 0 0 1 1 1 1
  line L137 (56.2422, 21.219) -> (56.3128, 21.1215) construction
  line L138 (56.3128, 21.1215) -> (56.3625, 20.9945) construction
  line L139 (56.3625, 20.9945) -> (56.3625, 20.9945) construction
  spline S44 degree 3 poles (56.3625, 20.9945) (56.3626, 20.9946) (56.411, 21.1216) (56.4821, 21.2186) knots 0 0 0 0 1 1 1 1
  line L140 (56.3625, 20.9945) -> (56.3625, 20.9945) construction
  line L141 (56.3625, 20.9945) -> (56.411, 21.1216) construction
  line L142 (56.411, 21.1216) -> (56.4821, 21.2186) construction
  spline S45 degree 3 poles (56.4821, 21.2186) (56.5192, 21.2695) (56.5642, 21.3176) (56.5642, 21.3863) knots 0 0 0 0 1 1 1 1
  line L143 (56.4821, 21.2186) -> (56.5192, 21.2695) construction
  line L144 (56.5192, 21.2695) -> (56.5642, 21.3176) construction
  line L145 (56.5642, 21.3176) -> (56.5642, 21.3863) construction
  spline S46 degree 3 poles (56.5642, 21.3863) (56.5642, 21.455) (56.52, 21.5023) (56.4825, 21.5532) knots 0 0 0 0 1 1 1 1
  line L146 (56.5642, 21.3863) -> (56.5642, 21.455) construction
  line L147 (56.5642, 21.455) -> (56.52, 21.5023) construction
  line L148 (56.52, 21.5023) -> (56.4825, 21.5532) construction
  spline S47 degree 3 poles (58.7522, 19.6166) (59.455, 19.7062) (60.2718, 19.8912) (60.7279, 19.4201) knots 0 0 0 0 1 1 1 1
  line L149 (58.7522, 19.6166) -> (59.455, 19.7062) construction
  line L150 (59.455, 19.7062) -> (60.2718, 19.8912) construction
  line L151 (60.2718, 19.8912) -> (60.7279, 19.4201) construction
  spline S48 degree 3 poles (60.7887, 19.7602) (60.6779, 21.18) (57.0275, 22.8574) (54.7435, 22.8167) knots 0 0 0 0 1 1 1 1
  line L152 (60.7887, 19.7602) -> (60.6779, 21.18) construction
  line L153 (60.6779, 21.18) -> (57.0275, 22.8574) construction
  line L154 (57.0275, 22.8574) -> (54.7435, 22.8167) construction
  spline S49 degree 3 poles (54.7435, 22.8167) (53.3905, 22.7914) (52.0915, 22.2963) (50.8205, 21.2139) knots 0 0 0 0 1 1 1 1
  line L155 (54.7435, 22.8167) -> (53.3905, 22.7914) construction
  line L156 (53.3905, 22.7914) -> (52.0915, 22.2963) construction
  line L157 (52.0915, 22.2963) -> (50.8205, 21.2139) construction
  spline S50 degree 3 poles (50.8205, 21.2139) (51.7253, 21.5757) (52.4928, 21.67) (53.1801, 21.6116) knots 0 0 0 0 1 1 1 1
  line L158 (50.8205, 21.2139) -> (51.7253, 21.5757) construction
  line L159 (51.7253, 21.5757) -> (52.4928, 21.67) construction
  line L160 (52.4928, 21.67) -> (53.1801, 21.6116) construction
  spline S51 degree 3 poles (53.1801, 21.6116) (50.4026, 20.4764) (50.3043, 17.7928) (50.3312, 17.056) knots 0 0 0 0 1 1 1 1
  line L161 (53.1801, 21.6116) -> (50.4026, 20.4764) construction
  line L162 (50.4026, 20.4764) -> (50.3043, 17.7928) construction
  line L163 (50.3043, 17.7928) -> (50.3312, 17.056) construction
  spline S52 degree 3 poles (50.3312, 17.056) (50.5344, 18.022) (51.0296, 18.8424) (51.8243, 19.5128) knots 0 0 0 0 1 1 1 1
  line L164 (50.3312, 17.056) -> (50.5344, 18.022) construction
  line L165 (50.5344, 18.022) -> (51.0296, 18.8424) construction
  line L166 (51.0296, 18.8424) -> (51.8243, 19.5128) construction
  spline S53 degree 3 poles (51.8243, 19.5128) (50.5794, 17.438) (50.5944, 15.0326) (52.0903, 13.4487) knots 0 0 0 0 1 1 1 1
  line L167 (51.8243, 19.5128) -> (50.5794, 17.438) construction
  line L168 (50.5794, 17.438) -> (50.5944, 15.0326) construction
  line L169 (50.5944, 15.0326) -> (52.0903, 13.4487) construction
  spline S54 degree 3 poles (52.0903, 13.4487) (52.2205, 13.3098) (52.3519, 13.1709) (52.4829, 13.0328) knots 0 0 0 0 1 1 1 1
  line L170 (52.0903, 13.4487) -> (52.2205, 13.3098) construction
  line L171 (52.2205, 13.3098) -> (52.3519, 13.1709) construction
  line L172 (52.3519, 13.1709) -> (52.4829, 13.0328) construction
  spline S55 degree 3 poles (52.4829, 13.0328) (51.7123, 15.1403) (52.183, 17.6152) (53.5144, 19.2405) knots 0 0 0 0 1 1 1 1
  line L173 (52.4829, 13.0328) -> (51.7123, 15.1403) construction
  line L174 (51.7123, 15.1403) -> (52.183, 17.6152) construction
  line L175 (52.183, 17.6152) -> (53.5144, 19.2405) construction
  line L176 (60.7279, 19.4201) -> (60.7887, 19.7602)
  spline S56 degree 3 poles (53.6221, 19.3707) (53.4654, 19.8344) (53.4047, 20.2187) (53.4493, 20.2396) knots 0 0 0 0 1 1 1 1
  line L177 (53.6221, 19.3707) -> (53.4654, 19.8344) construction
  line L178 (53.4654, 19.8344) -> (53.4047, 20.2187) construction
  line L179 (53.4047, 20.2187) -> (53.4493, 20.2396) construction
  spline S57 degree 3 poles (53.4493, 20.2396) (53.7026, 19.847) (53.9492, 19.4516) (54.2408, 19.1024) knots 0 0 0 0 1 1 1 1
  line L180 (53.4493, 20.2396) -> (53.7026, 19.847) construction
  line L181 (53.7026, 19.847) -> (53.9492, 19.4516) construction
  line L182 (53.9492, 19.4516) -> (54.2408, 19.1024) construction
  spline S58 degree 3 poles (54.2408, 19.1024) (54.6694, 18.591) (55.1977, 18.1787) (55.992, 18.011) knots 0 0 0 0 1 1 1 1
  line L183 (54.2408, 19.1024) -> (54.6694, 18.591) construction
  line L184 (54.6694, 18.591) -> (55.1977, 18.1787) construction
  line L185 (55.1977, 18.1787) -> (55.992, 18.011) construction
  spline S59 degree 3 poles (55.992, 18.011) (57.8624, 18.5271) (59.3078, 18.2801) (59.5829, 18.3389) knots 0 0 0 0 1 1 1 1
  line L186 (55.992, 18.011) -> (57.8624, 18.5271) construction
  line L187 (57.8624, 18.5271) -> (59.3078, 18.2801) construction
  line L188 (59.3078, 18.2801) -> (59.5829, 18.3389) construction
  spline S60 degree 3 poles (59.5829, 18.3389) (59.5939, 18.3429) (59.6038, 18.3459) (59.616, 18.3499) knots 0 0 0 0 1 1 1 1
  line L189 (59.5829, 18.3389) -> (59.5939, 18.3429) construction
  line L190 (59.5939, 18.3429) -> (59.6038, 18.3459) construction
  line L191 (59.6038, 18.3459) -> (59.616, 18.3499) construction
  spline S61 degree 3 poles (59.616, 18.3499) (60.0654, 18.4576) (60.3325, 18.6371) (60.5338, 18.8423) knots 0 0 0 0 1 1 1 1
  line L192 (59.616, 18.3499) -> (60.0654, 18.4576) construction
  line L193 (60.0654, 18.4576) -> (60.3325, 18.6371) construction
  line L194 (60.3325, 18.6371) -> (60.5338, 18.8423) construction
  spline S62 degree 3 poles (60.5338, 18.8423) (60.1072, 19.1454) (59.5248, 19.1051) (58.8244, 19.0167) knots 0 0 0 0 1 1 1 1
  line L195 (60.5338, 18.8423) -> (60.1072, 19.1454) construction
  line L196 (60.1072, 19.1454) -> (59.5248, 19.1051) construction
  line L197 (59.5248, 19.1051) -> (58.8244, 19.0167) construction
  spline S63 degree 3 poles (58.8244, 19.0167) (56.8001, 18.7603) (56.2374, 19.2405) (55.2679, 20.2388) knots 0 0 0 0 1 1 1 1
  line L198 (58.8244, 19.0167) -> (56.8001, 18.7603) construction
  line L199 (56.8001, 18.7603) -> (56.2374, 19.2405) construction
  line L200 (56.2374, 19.2405) -> (55.2679, 20.2388) construction
  spline S64 degree 3 poles (55.2679, 20.2388) (55.3318, 20.2183) (57.5664, 19.4654) (58.7522, 19.6165) knots 0 0 0 0 1 1 1 1
  line L201 (55.2679, 20.2388) -> (55.3318, 20.2183) construction
  line L202 (55.3318, 20.2183) -> (57.5664, 19.4654) construction
  line L203 (57.5664, 19.4654) -> (58.7522, 19.6165) construction
  line L204 (53.5144, 19.2405) -> (53.6221, 19.3707)
  spline S65 degree 3 poles (56.9493, 21.2376) (56.9453, 21.221) (56.9403, 21.2033) (56.9351, 21.1867) knots 0 0 0 0 1 1 1 1
  line L205 (56.9493, 21.2376) -> (56.9453, 21.221) construction
  line L206 (56.9453, 21.221) -> (56.9403, 21.2033) construction
  line L207 (56.9403, 21.2033) -> (56.9351, 21.1867) construction
  spline S66 degree 3 poles (56.9351, 21.1867) (56.9251, 21.1559) (56.913, 21.1271) (56.8988, 21.0995) knots 0 0 0 0 1 1 1 1
  line L208 (56.9351, 21.1867) -> (56.9251, 21.1559) construction
  line L209 (56.9251, 21.1559) -> (56.913, 21.1271) construction
  line L210 (56.913, 21.1271) -> (56.8988, 21.0995) construction
  spline S67 degree 3 poles (56.8988, 21.0995) (56.8948, 21.0925) (56.8918, 21.0861) (56.8882, 21.0802) knots 0 0 0 0 1 1 1 1
  line L211 (56.8988, 21.0995) -> (56.8948, 21.0925) construction
  line L212 (56.8948, 21.0925) -> (56.8918, 21.0861) construction
  line L213 (56.8918, 21.0861) -> (56.8882, 21.0802) construction
  spline S68 degree 3 poles (56.8882, 21.0802) (56.8772, 21.0593) (56.8645, 21.0392) (56.8515, 21.0194) knots 0 0 0 0 1 1 1 1
  line L214 (56.8882, 21.0802) -> (56.8772, 21.0593) construction
  line L215 (56.8772, 21.0593) -> (56.8645, 21.0392) construction
  line L216 (56.8645, 21.0392) -> (56.8515, 21.0194) construction
  spline S69 degree 3 poles (56.8515, 21.0194) (56.8455, 21.0124) (56.8405, 21.0044) (56.8353, 20.9973) knots 0 0 0 0 1 1 1 1
  line L217 (56.8515, 21.0194) -> (56.8455, 21.0124) construction
  line L218 (56.8455, 21.0124) -> (56.8405, 21.0044) construction
  line L219 (56.8405, 21.0044) -> (56.8353, 20.9973) construction
  spline S70 degree 3 poles (56.8353, 20.9973) (56.8263, 20.9863) (56.8183, 20.9764) (56.8093, 20.9653) knots 0 0 0 0 1 1 1 1
  line L220 (56.8353, 20.9973) -> (56.8263, 20.9863) construction
  line L221 (56.8263, 20.9863) -> (56.8183, 20.9764) construction
  line L222 (56.8183, 20.9764) -> (56.8093, 20.9653) construction
  spline S71 degree 3 poles (56.8093, 20.9653) (56.7963, 20.9519) (56.784, 20.9385) (56.7714, 20.9266) knots 0 0 0 0 1 1 1 1
  line L223 (56.8093, 20.9653) -> (56.7963, 20.9519) construction
  line L224 (56.7963, 20.9519) -> (56.784, 20.9385) construction
  line L225 (56.784, 20.9385) -> (56.7714, 20.9266) construction
  spline S72 degree 3 poles (56.7714, 20.9266) (56.7624, 20.9186) (56.7533, 20.9104) (56.7442, 20.9021) knots 0 0 0 0 1 1 1 1
  line L226 (56.7714, 20.9266) -> (56.7624, 20.9186) construction
  line L227 (56.7624, 20.9186) -> (56.7533, 20.9104) construction
  line L228 (56.7533, 20.9104) -> (56.7442, 20.9021) construction
  spline S73 degree 3 poles (56.7442, 20.9021) (56.7312, 20.8911) (56.7186, 20.8816) (56.7047, 20.8729) knots 0 0 0 0 1 1 1 1
  line L229 (56.7442, 20.9021) -> (56.7312, 20.8911) construction
  line L230 (56.7312, 20.8911) -> (56.7186, 20.8816) construction
  line L231 (56.7186, 20.8816) -> (56.7047, 20.8729) construction
  spline S74 degree 3 poles (56.7047, 20.8729) (56.6941, 20.8649) (56.683, 20.8579) (56.6731, 20.8508) knots 0 0 0 0 1 1 1 1
  line L232 (56.7047, 20.8729) -> (56.6941, 20.8649) construction
  line L233 (56.6941, 20.8649) -> (56.683, 20.8579) construction
  line L234 (56.683, 20.8579) -> (56.6731, 20.8508) construction
  spline S75 degree 3 poles (56.6731, 20.8508) (56.6581, 20.8418) (56.6435, 20.8338) (56.6285, 20.8259) knots 0 0 0 0 1 1 1 1
  line L235 (56.6731, 20.8508) -> (56.6581, 20.8418) construction
  line L236 (56.6581, 20.8418) -> (56.6435, 20.8338) construction
  line L237 (56.6435, 20.8338) -> (56.6285, 20.8259) construction
  spline S76 degree 3 poles (56.6285, 20.8259) (56.6225, 20.8229) (56.6151, 20.8199) (56.6092, 20.8159) knots 0 0 0 0 1 1 1 1
  line L238 (56.6285, 20.8259) -> (56.6225, 20.8229) construction
  line L239 (56.6225, 20.8229) -> (56.6151, 20.8199) construction
  line L240 (56.6151, 20.8199) -> (56.6092, 20.8159) construction
  spline S77 degree 3 poles (56.6092, 20.8159) (56.5824, 20.8045) (56.554, 20.7938) (56.5259, 20.7851) knots 0 0 0 0 1 1 1 1
  line L241 (56.6092, 20.8159) -> (56.5824, 20.8045) construction
  line L242 (56.5824, 20.8045) -> (56.554, 20.7938) construction
  line L243 (56.554, 20.7938) -> (56.5259, 20.7851) construction
  line L244 (56.9513, 21.2376) -> (56.9493, 21.2376)
  spline S78 degree 3 poles (56.525, 20.7851) (56.5021, 20.7791) (56.4788, 20.7741) (56.4551, 20.7701) knots 0 0 0 0 1 1 1 1
  line L245 (56.525, 20.7851) -> (56.5021, 20.7791) construction
  line L246 (56.5021, 20.7791) -> (56.4788, 20.7741) construction
  line L247 (56.4788, 20.7741) -> (56.4551, 20.7701) construction
  spline S79 degree 3 poles (56.4551, 20.7701) (56.4501, 20.7693) (56.4451, 20.7681) (56.4389, 20.7681) knots 0 0 0 0 1 1 1 1
  line L248 (56.4551, 20.7701) -> (56.4501, 20.7693) construction
  line L249 (56.4501, 20.7693) -> (56.4451, 20.7681) construction
  line L250 (56.4451, 20.7681) -> (56.4389, 20.7681) construction
  spline S80 degree 3 poles (56.4389, 20.7681) (56.4137, 20.7641) (56.3888, 20.7621) (56.3631, 20.7621) knots 0 0 0 0 1 1 1 1
  line L251 (56.4389, 20.7681) -> (56.4137, 20.7641) construction
  line L252 (56.4137, 20.7641) -> (56.3888, 20.7621) construction
  line L253 (56.3888, 20.7621) -> (56.3631, 20.7621) construction
  line L254 (56.5259, 20.7851) -> (56.525, 20.7851)
  spline S81 degree 3 poles (56.3551, 20.7621) (56.3306, 20.7629) (56.307, 20.7641) (56.2829, 20.7681) knots 0 0 0 0 1 1 1 1
  line L255 (56.3551, 20.7621) -> (56.3306, 20.7629) construction
  line L256 (56.3306, 20.7629) -> (56.307, 20.7641) construction
  line L257 (56.307, 20.7641) -> (56.2829, 20.7681) construction
  spline S82 degree 3 poles (56.2829, 20.7681) (56.2769, 20.7681) (56.2726, 20.7691) (56.2671, 20.7701) knots 0 0 0 0 1 1 1 1
  line L258 (56.2829, 20.7681) -> (56.2769, 20.7681) construction
  line L259 (56.2769, 20.7681) -> (56.2726, 20.7691) construction
  line L260 (56.2726, 20.7691) -> (56.2671, 20.7701) construction
  spline S83 degree 3 poles (56.2671, 20.7701) (56.2422, 20.7741) (56.219, 20.7791) (56.1953, 20.7863) knots 0 0 0 0 1 1 1 1
  line L261 (56.2671, 20.7701) -> (56.2422, 20.7741) construction
  line L262 (56.2422, 20.7741) -> (56.219, 20.7791) construction
  line L263 (56.219, 20.7791) -> (56.1953, 20.7863) construction
  line L264 (56.3631, 20.7621) -> (56.3551, 20.7621)
  spline S84 degree 3 poles (56.1903, 20.7883) (56.1635, 20.7963) (56.1382, 20.8065) (56.1133, 20.8171) knots 0 0 0 0 1 1 1 1
  line L265 (56.1903, 20.7883) -> (56.1635, 20.7963) construction
  line L266 (56.1635, 20.7963) -> (56.1382, 20.8065) construction
  line L267 (56.1382, 20.8065) -> (56.1133, 20.8171) construction
  spline S85 degree 3 poles (56.1133, 20.8171) (56.1103, 20.8191) (56.1083, 20.8211) (56.1053, 20.8221) knots 0 0 0 0 1 1 1 1
  line L268 (56.1133, 20.8171) -> (56.1103, 20.8191) construction
  line L269 (56.1103, 20.8191) -> (56.1083, 20.8211) construction
  line L270 (56.1083, 20.8211) -> (56.1053, 20.8221) construction
  spline S86 degree 3 poles (56.1053, 20.8221) (56.0832, 20.8321) (56.0611, 20.8442) (56.0402, 20.8584) knots 0 0 0 0 1 1 1 1
  line L271 (56.1053, 20.8221) -> (56.0832, 20.8321) construction
  line L272 (56.0832, 20.8321) -> (56.0611, 20.8442) construction
  line L273 (56.0611, 20.8442) -> (56.0402, 20.8584) construction
  spline S87 degree 3 poles (56.0402, 20.8584) (56.0372, 20.8604) (56.0342, 20.8614) (56.0322, 20.8634) knots 0 0 0 0 1 1 1 1
  line L274 (56.0402, 20.8584) -> (56.0372, 20.8604) construction
  line L275 (56.0372, 20.8604) -> (56.0342, 20.8614) construction
  line L276 (56.0342, 20.8614) -> (56.0322, 20.8634) construction
  spline S88 degree 3 poles (56.0322, 20.8634) (56.0101, 20.878) (55.9892, 20.8938) (55.9695, 20.9119) knots 0 0 0 0 1 1 1 1
  line L277 (56.0322, 20.8634) -> (56.0101, 20.878) construction
  line L278 (56.0101, 20.878) -> (55.9892, 20.8938) construction
  line L279 (55.9892, 20.8938) -> (55.9695, 20.9119) construction
  spline S89 degree 3 poles (55.9695, 20.9119) (55.9655, 20.9149) (55.9625, 20.9179) (55.9595, 20.9219) knots 0 0 0 0 1 1 1 1
  line L280 (55.9695, 20.9119) -> (55.9655, 20.9149) construction
  line L281 (55.9655, 20.9149) -> (55.9625, 20.9179) construction
  line L282 (55.9625, 20.9179) -> (55.9595, 20.9219) construction
  spline S90 degree 3 poles (55.9595, 20.9219) (55.9422, 20.9369) (55.9264, 20.9535) (55.9114, 20.9708) knots 0 0 0 0 1 1 1 1
  line L283 (55.9595, 20.9219) -> (55.9422, 20.9369) construction
  line L284 (55.9422, 20.9369) -> (55.9264, 20.9535) construction
  line L285 (55.9264, 20.9535) -> (55.9114, 20.9708) construction
  spline S91 degree 3 poles (55.9114, 20.9708) (55.9084, 20.9738) (55.9044, 20.9778) (55.9014, 20.9815) knots 0 0 0 0 1 1 1 1
  line L286 (55.9114, 20.9708) -> (55.9084, 20.9738) construction
  line L287 (55.9084, 20.9738) -> (55.9044, 20.9778) construction
  line L288 (55.9044, 20.9778) -> (55.9014, 20.9815) construction
  spline S92 degree 3 poles (55.9014, 20.9815) (55.8844, 21.002) (55.8694, 21.0241) (55.8552, 21.0458) knots 0 0 0 0 1 1 1 1
  line L289 (55.9014, 20.9815) -> (55.8844, 21.002) construction